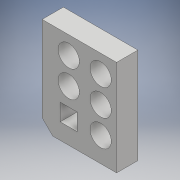
# Autodesk Inventor part: Contact
Saved by Autodesk Inventor 2018 (Build 220112000, 112)
## iProperties
Created: 2020-05-15
Part Number: Contact
Material: Generic
Document SubType Name: Modeling
Designer: Сергей
Density: 1 g/cm^3
Appearance: Default
Author: Сергей
Autodesk Inventor part; units mm, degrees
ref_plane "YZ Plane" through (0, 0, 0) normal (1, 0, 0) x (0, 1, 0)
ref_plane "XZ Plane" through (0, 0, 0) normal (0, 1, 0) x (-1, 0, 0)
ref_plane "XY Plane" through (0, 0, 0) normal (0, 0, 1) x (1, 0, 0)
sketch "Sketch1" plane through (0, 0, 0) normal (0, 1, 0) x (-1, 0, 0)
  line L0 (0, 0) -> (-7, 0)
  line L1 (-7, 0) -> (-7, -9)
  line L2 (-7, -9) -> (-1, -9)
  line L3 (0, 0) -> (0, -8)
  line L4 (0, -8) -> (-1, -9)
  dimension "d0" = 7
  dimension "d1" = 9
  dimension "d2" = 6
  dimension "d3" = 8
  constraints: 10 end point, 2 perpendicular, 1 horizontal, 1 vertical
  measures "d0" distance of L0.start L0.end
  measures "d1" distance of L0.end L1.end
  measures "d2" distance of L1.end L2.end
  measures "d3" distance of L0.start L3.end
extrude "Extrusion1" add sketch "Sketch1" along normal mid plane 2
hole "Hole1" at (5.5006, 1, -1.6898) direction (0, 1, 0) diameter 2 end through all both
pattern_linear "Rectangular Pattern1" count 3 spacing 2.5 along (0, 0, -1) of "Hole1"
pattern_linear "Rectangular Pattern2" count 2 spacing 3 along (-1, 0, 0) of "Hole1"
pattern_linear "Rectangular Pattern3" count 2 spacing 2.5 along (0, 0, -1) of "Rectangular Pattern2"
sketch "Sketch4" plane through (0, 0, 0) normal (0, 1, 0) x (-1, 0, 0)
  line L0 (0, -8) -> (0, 0) projected
  line L1 (-1.7006, -5.8898) -> (-3.3006, -5.8898)
  line L2 (-3.3006, -5.8898) -> (-3.3006, -7.4898)
  line L3 (-3.3006, -7.4898) -> (-1.7006, -7.4898)
  line L4 (-1.7006, -7.4898) -> (-1.7006, -5.8898)
  line L5 (-1.7006, -5.8898) -> (-3.3006, -7.4898) construction
  line L6 (-3.3006, -5.8898) -> (-1.7006, -7.4898) construction
  point P0 (-2.5006, -6.6898)
  dimension "d73" = 1.6
  dimension "d74" = 1.6
  constraints: 12 end point, 2 midpoint, 2 parallel, 1 horizontal, 1 perpendicular
  measures "d73" distance of L3.end L2.end
  measures "d74" distance of L2.end L1.end
extrude "Extrusion3" add sketch "Sketch4" along normal mid plane 2.1 separate body
combine bodies "Combine1" operation type subtract main body 1 bodies to subtract 2
body "Solid1"
